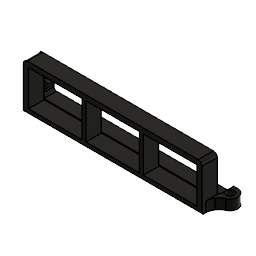
Main Switch Holder V1 (Autodesk Fusion 360 design; units mm, degrees)
part number: 2026-03-23-21-44-21-721
Autodesk Fusion 360 part; units mm, degrees
sketch "Sketch1" plane through (0, 0, 0) normal (0, 0, 1) x (1, 0, 0)
  line L0 (35, 9) -> (-35, 9)
  line L1 (-35, 9) -> (-35, -9)
  line L2 (-35, -9) -> (35, -9)
  line L3 (35, -9) -> (35, 9)
  line L4 (35, 9) -> (-35, -9) construction
  line L5 (-35, 9) -> (35, -9) construction
  line L6 (10.5, 7) -> (-10.5, 7) construction
  line L7 (-10.5, 7) -> (-10.5, -7) construction
  line L8 (-10.5, -7) -> (10.5, -7) construction
  line L9 (10.5, -7) -> (10.5, 7) construction
  line L10 (10.5, 7) -> (-10.5, -7) construction
  line L11 (-10.5, 7) -> (10.5, -7) construction
  line L12 (10.5, 7) -> (-10.5, 7)
  line L13 (-10.5, 7) -> (-10.5, -7)
  line L14 (-10.5, -7) -> (10.5, -7)
  line L15 (10.5, -7) -> (10.5, 7)
  line L16 (10.5, 7) -> (-10.5, -7) construction
  line L17 (-10.5, 7) -> (10.5, -7) construction
  line L18 (0, 0) -> (-22.5, 0)
  line L19 (-12, 7) -> (-33, 7) construction
  line L20 (-33, 7) -> (-33, -7) construction
  line L21 (-33, -7) -> (-12, -7) construction
  line L22 (-12, -7) -> (-12, 7) construction
  line L23 (-12, 7) -> (-33, -7) construction
  line L24 (-33, 7) -> (-12, -7) construction
  line L25 (-12, -7) -> (-33, -7)
  line L26 (-33, -7) -> (-33, 7)
  line L27 (-33, 7) -> (-12, 7)
  line L28 (-12, 7) -> (-12, -7)
  line L29 (-12, -7) -> (-33, 7) construction
  line L30 (-33, -7) -> (-12, 7) construction
  line L31 (0, 9) -> (0, -9) construction
  line L32 (33, 7) -> (12, 7)
  line L33 (33, -7) -> (33, 7)
  line L34 (33, 7) -> (33, -7) construction
  line L35 (12, 7) -> (33, 7) construction
  line L36 (12, -7) -> (12, 7) construction
  line L37 (33, -7) -> (12, -7) construction
  line L38 (12, -7) -> (33, -7)
  line L39 (12, 7) -> (12, -7)
  point P0 (-22.5, 0)
  point P1 (-22.5, 0)
  dimension "d1" = 70
  dimension "d2" = 18
  dimension "d3" = 21
  dimension "d4" = 14
  dimension "d8" = 21
  dimension "d9" = 14
  dimension "d10" = 22.5
  dimension "d11" = 21
  dimension "d12" = 14
  dimension "d13" = 21
  dimension "d14" = 14
  constraint horizontal L0
  constraint perpendicular L0 L1
  constraint parallel L0 L2
  constraint parallel L1 L3
  constraint coincident L4 L18.start
  constraint coincident L5 L18.start
  constraint coincident L18.start origin
  constraint horizontal L6
  constraint perpendicular L6 L7
  constraint parallel L6 L8
  constraint parallel L7 L9
  constraint coincident L10 L18.start
  constraint coincident L11 L18.start
  constraint horizontal L12
  constraint perpendicular L12 L13
  constraint parallel L12 L14
  constraint parallel L13 L15
  constraint coincident L16 L18.start
  constraint coincident L17 L18.start
  constraint horizontal L18
  constraint horizontal L19
  constraint perpendicular L19 L20
  constraint parallel L19 L21
  constraint parallel L20 L22
  constraint coincident L23 P1
  constraint coincident L24 P1
  constraint coincident P1 P0
  constraint horizontal L25
  constraint perpendicular L25 L26
  constraint parallel L25 L27
  constraint parallel L26 L28
  constraint coincident L29 P1
  constraint coincident L30 P1
  constraint midpoint L0 L31.start
  constraint midpoint L2 L31.end
  constraint symmetric L19.start L31 L32.end
  constraint symmetric L19.end L31 L32.start
  constraint symmetric L20.end L31 L33.start
  constraint symmetric L21.end L31 L36.start
  measures "d1" distance of L1.end L2.end
  measures "d2" distance of L0.end L1.end
  measures "d3" distance of L7.end L8.end
  measures "d4" distance of L6.end L7.end
  measures "d8" distance of L7.end L8.end
  measures "d9" distance of L6.end L7.end
  measures "d10" distance of L18.start P1
  measures "d11" distance of L20.end L21.end
  measures "d12" distance of L19.end L20.end
  measures "d13" distance of L19.end L19.start
  measures "d14" distance of L20.end L19.end
extrude "Extrude4" add sketch "Sketch1" along normal blind 6
sketch "Sketch3" plane through (0, -9, 0) normal (0, -1, 0) x (1, 0, 0)
  line L0 (-35, 0) -> (35, 0)
  line L1 (35, 0) -> (35, 6)
  line L2 (35, 6) -> (-35, 6)
  line L3 (-35, 6) -> (-35, 0)
  line L4 (-35, 0) -> (35, 0)
  line L5 (0, 0) -> (0, -3)
  line L6 (-37, -3) -> (37, -3)
  circle A0 centre (-37, -3) radius 1.65
  circle A1 centre (37, -3) radius 1.65
  circle A2 centre (37, -3) radius 3
  circle A3 centre (-37, -3) radius 3
  line L7 (-35, 0) -> (-37, 0)
  line L8 (35, 0) -> (37, 0)
  line L9 (37, -6) -> (-37, -6)
  line L10 (35, 3) -> (37, 0)
  line L11 (-35, 3) -> (-37, 0)
  line L12 (35, 0) -> (35, -0.7639)
  line L13 (-35, 0) -> (-35, -0.7639)
  dimension "d43" = 3
  dimension "d44" = 74
  dimension "d45" = 3.3
  dimension "d46" = 3.3
  dimension "d47" = 6
  dimension "d48" = 6
  constraint coincident L0.start L3.end
  constraint coincident L0.end L1.start
  constraint coincident L5.start origin
  constraint perpendicular L4 L5
  constraint midpoint L5.end L6
  constraint perpendicular L5 L6
  constraint coincident L6.start A0.centre
  constraint coincident L6.end A1.centre
  constraint concentric A1 A2
  constraint concentric A0 A3
  constraint coincident A3 L7.end
  constraint tangent A3 L7
  constraint coincident A2 L8.end
  constraint tangent A2 L8
  constraint coincident A2 L9.start
  constraint coincident A3 L9.end
  constraint tangent A3 L9
  constraint parallel L6 L9
  constraint midpoint L1 L10.start
  constraint midpoint L3 L11.start
  constraint coincident A2 L12.end
  constraint perpendicular L4 L12
  constraint coincident A3 L13.end
  constraint perpendicular L4 L13
  measures "d43" distance of L5.start L5.end
  measures "d44" distance of L6.start L6.end
  measures "d45" diameter of A0
  measures "d46" diameter of A1
  measures "d47" diameter of A2
  measures "d48" diameter of A3
extrude "Extrude9" add sketch "Sketch3" against normal blind 4 contours L3 L7 L11 | A3 L7 L13 | L0 L4 L5 L6 A3 L13 | L0 L4 L5 L6 A2 L12 | A3 | L1 L8 L10 | A2 L8 L12 | L6 A2 A3 L9 | A2
sketch "Sketch5" plane through (0, -5, 0) normal (0, 1, 0) x (-1, 0, 0)
  circle A0 centre (37, -3) radius 1.65
  circle A1 centre (-37, -3) radius 1.65
  line L0 (35, 3) -> (35, 0)
  line L1 (35, 0) -> (33, 0)
  line L2 (33, 0) -> (12, 0)
  line L3 (12, 0) -> (10.5, 0)
  line L4 (10.5, 0) -> (-10.5, 0)
  line L5 (-10.5, 0) -> (-12, 0)
  line L6 (-12, 0) -> (-33, 0)
  line L7 (-33, 0) -> (-35, 0)
  line L8 (-35, 0) -> (-35, 3)
  line L9 (-35, 3) -> (-37, 0)
  arc A2 (-37, 0) -> (-37, -6) centre (-37, -3) ccw
  line L10 (-37, -6) -> (37, -6)
  arc A3 (37, -6) -> (37, 0) centre (37, -3) ccw
  line L11 (37, 0) -> (35, 3)
  line L12 (-35, 0) -> (35, 0)
  line L13 (35, 0) -> (35, -6)
  line L14 (35, -6) -> (-35, -6)
  line L15 (-35, -6) -> (-35, 0)
  dimension "d67" = 70
  dimension "d68" = 6
  constraint horizontal L12
  constraint vertical L13
  constraint horizontal L14
  constraint vertical L15
  constraint coincident L7.end L8.start
  measures "d67" distance of L7.end L0.end
  measures "d68" distance of L7.end L14.end
extrude "Extrude10" cut sketch "Sketch5" against normal blind 2.5 contours L1 L2 L3 L4 L5 L6 L7 L10 L12 L13 L14 L15
fillet "Fillet10" radius 5 4 edges at (-35, -7, 3) (-37, -7, 0) (37, -7, 0) (35, -7, 3)
fillet "Fillet11" radius 1.75 2 edges at (35, -6.25, 0) (-35, -6.25, 0)
fillet "Fillet12" radius 1 4 edges at (-34.4874, -7.5, -0.5126) (-35, -7.5, -3.875) (35, -7.5, -3.875) (34.4874, -7.5, -0.5126)
fillet "Fillet13" radius 0.5 4 edges at (35, -5, -3.875) (34.4874, -5, -0.5126) (-34.4874, -5, -0.5126) (-35, -5, -3.875)
fillet "Fillet14" radius 1.5 2 edges at (-35, 9, 3) (35, 9, 3)
fillet "Fillet15" radius 0.5 1 edges at (0, -9, 6)
extrude "Extrude1" [suppressed]
sketch "Sketch2" plane through (0, -9, 0) normal (0, -1, 0) x (1, 0, 0)
  line L0 (-35, 0) -> (35, 0)
  line L1 (35, 0) -> (35, 8)
  line L2 (35, 8) -> (-35, 8)
  line L3 (-35, 8) -> (-35, 0)
  line L4 (0, 0) -> (0, 4)
  line L5 (-36, 4) -> (36, 4)
  circle A0 centre (36, 4) radius 1.65
  circle A1 centre (-36, 4) radius 1.65
  line L6 (-35, 8) -> (-41, 8)
  line L7 (-41, 8) -> (-41, 0)
  line L8 (-41, 0) -> (-35, 0)
  line L9 (-35, 0) -> (-35, 8)
  line L10 (35, 8) -> (41, 8)
  line L11 (41, 8) -> (41, 0)
  line L12 (41, 0) -> (35, 0)
  line L13 (35, 0) -> (35, 8)
  dimension "d17" = 72
  dimension "d18" = 3.3
  dimension "d19" = 3.3
  dimension "d21" = 6
  dimension "d22" = 8
  dimension "d23" = 6
  dimension "d24" = 8
  constraint coincident L4.start origin
  constraint perpendicular L0 L4
  constraint midpoint L4.end L5
  constraint perpendicular L1 L5
  constraint coincident L5.end A0.centre
  constraint coincident L5.start A1.centre
  constraint coincident L2.end L3.start
  constraint horizontal L6
  constraint vertical L7
  constraint horizontal L8
  constraint vertical L9
  constraint horizontal L10
  constraint vertical L11
  constraint horizontal L12
  constraint vertical L13
  constraint coincident L1.end L2.start
  measures "d17" distance of L5.start L5.end
  measures "d18" diameter of A0
  measures "d19" diameter of A1
  measures "d21" distance of L2.end L6.end
  measures "d22" distance of L2.end L0.start
  measures "d23" distance of L1.end L10.end
  measures "d24" distance of L1.end L0.end
extrude "Extrude2" [suppressed]
fillet "Fillet1" [suppressed]
fillet "Fillet2" [suppressed]
fillet "Fillet3" [suppressed]
extrude "Extrude3" [suppressed]
fillet "Fillet4" [suppressed]
fillet "Fillet5" [suppressed]
fillet "Fillet6" [suppressed]
